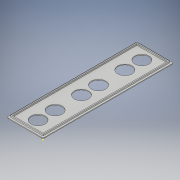
# Autodesk Inventor part: nixielid
Saved by Autodesk Inventor 2019 (Build 230136000, 136)
## iProperties
Created: 2023-02-11
Part Number: nixielid
Material: Generic
Document SubType Name: Modeling
Designer: Matt
Density: 1 g/cm^3
Appearance: Default
Author: Matt
Autodesk Inventor part; units mm, degrees
ref_plane "YZ Plane" through (0, 0, 0) normal (1, 0, 0) x (0, 1, 0)
ref_plane "XZ Plane" through (0, 0, 0) normal (0, 1, 0) x (-1, 0, 0)
ref_plane "XY Plane" through (0, 0, 0) normal (0, 0, 1) x (1, 0, 0)
sketch "Sketch1" plane through (0, 0, 0) normal (0, 1, 0) x (-1, 0, 0)
  line L0 (0, 0) -> (51, 0)
  line L1 (51, 0) -> (51, -183)
  line L2 (51, -183) -> (0, -183)
  line L3 (0, -183) -> (0, 0)
  line L4 (2.5, -2.5) -> (48.5, -2.5)
  line L5 (48.5, -2.5) -> (48.5, -180.5)
  line L6 (48.5, -180.5) -> (2.5, -180.5)
  line L7 (2.5, -180.5) -> (2.5, -2.5)
  line L8 (2.5, -2.5) -> (48.5, -180.5) construction
  line L9 (48.5, -2.5) -> (2.5, -180.5) construction
  point P0 (25.5, -91.5)
  dimension "d0" = 51
  dimension "d1" = 183
  dimension "d2" = 46
  dimension "d3" = 178
  dimension "d4" = 2.5
  dimension "d5" = 2.5
  constraints: 20 end point, 4 parallel, 2 horizontal, 2 midpoint, 2 perpendicular
  measures "d0" distance of L1.end L2.end
  measures "d1" distance of L0.end L1.end
  measures "d2" distance of L5.end L6.end
  measures "d3" distance of L4.end L5.end
  measures "d4" distance between parallel lines of L0 L4
  measures "d5" distance between parallel lines of L1 L5
extrude "Extrusion1" add sketch "Sketch1" along normal blind 2
extrude "Extrusion2" add sketch "Sketch1" along normal blind 4 contours L4 L5 L6 L7
sketch "Sketch2" plane through (0, 4, 0) normal (0, 1, 0) x (1, 0, 0)
  point P0 (0, 0)
sketch "Sketch3" plane through (0, 4, 0) normal (0, 1, 0) x (1, 0, 0)
  line L0 (-47, 4) -> (-4, 4)
  line L1 (-4, 4) -> (-4, 179)
  line L2 (-4, 179) -> (-47, 179)
  line L3 (-47, 179) -> (-47, 4)
  line L4 (-47, 4) -> (-4, 179) construction
  line L5 (-4, 4) -> (-47, 179) construction
  line L6 (-48.5, 2.5) -> (-2.5, 2.5) projected
  line L7 (-48.5, 180.5) -> (-48.5, 2.5) projected
  point P0 (0, 0)
  point P1 (-25.5, 91.5)
  dimension "d10" = 43
  dimension "d11" = 175
  dimension "d12" = 1.5
  dimension "d13" = 1.5
  constraints: 12 end point, 2 midpoint, 2 parallel, 1 horizontal, 1 perpendicular
  measures "d10" distance of L2.end L1.end
  measures "d11" distance of L1.end L0.end
  measures "d12" distance between parallel lines of L6 L0
  measures "d13" distance between parallel lines of L7 L3
extrude "Extrusion3" cut sketch "Sketch3" against normal blind 2
sketch "Sketch4" plane through (0, 0, 0) normal (0, -1, 0) x (1, 0, 0)
  point P0 (0, 0)
sketch "Sketch5" plane through (0, 0, 0) normal (0, -1, 0) x (1, 0, 0)
  circle A0 centre (-25.5, -18.5) radius 10
  circle A1 centre (-25.5, -42.5) radius 10
  circle A2 centre (-25.5, -79.5) radius 10
  circle A3 centre (-25.5, -103.5) radius 10
  circle A4 centre (-25.5, -140.5) radius 10
  circle A5 centre (-25.5, -164.5) radius 10
  point P0 (0, 0)
  dimension "d16" = 20
  dimension "d17" = 20
  dimension "d18" = 20
  dimension "d19" = 20
  dimension "d20" = 20
  dimension "d21" = 20
  constraints: 6 centre point
  measures "d16" diameter of A0
  measures "d17" diameter of A1
  measures "d18" diameter of A2
  measures "d19" diameter of A3
  measures "d20" diameter of A4
  measures "d21" diameter of A5
sketch "Sketch6" plane through (0, 0, 0) normal (0, -1, 0) x (1, 0, 0)
  point P0 (0, 0)
extrude "Extrusion4" cut sketch "Sketch5" against normal blind 5
fillet "Fillet1" radius 2 4 edges at (-51, 1, 0) (-51, 1, -183) (0, 1, -183) (0, 1, 0)
fillet "Fillet2" radius 1 6 edges at (-35.5, 0, -103.5) (-35.5, 0, -79.5) (-35.5, 0, -42.5) (-35.5, 0, -18.5) (-35.5, 0, -140.5) (-35.5, 0, -164.5)
fillet "Fillet3" radius 1 8 edges at (-50.4142, 0, -182.4142) (-25.5, 0, -183) (-0.5858, 0, -182.4142) (0, 0, -91.5) (-0.5858, 0, -0.5858) (-25.5, 0, 0) (-50.4142, 0, -0.5858) (-51, 0, -91.5)
body "Solid1"
